Autodesk Fusion 360 part; units mm, degrees
note: some values were not read from the file. Set by a fixed rule: which sketch regions a step uses.
(part 17 of 59)
  spline S95 degree 5 poles (2.1183, -16.4679) (2.1183, -16.468) (2.1183, -16.4682) (2.1183, -16.4685) (2.1184, -16.469) (2.1184, -16.4698) (2.1185, -16.4706) (2.1186, -16.4716) (2.1187, -16.4727) (2.1188, -16.4739) (2.1189, -16.4752) (2.1191, -16.4766) (2.1192, -16.4781) (2.1194, -16.4798) (2.1196, -16.4815) (2.1198, -16.4833) (2.12, -16.4852) (2.1202, -16.4873) (2.1204, -16.4894) (2.1207, -16.4916) (2.121, -16.4939) (2.1212, -16.4963) (2.1215, -16.4989) (2.1219, -16.5015) (2.1222, -16.5041) (2.1225, -16.5069) (2.1229, -16.5098) (2.1233, -16.5128) (2.1237, -16.5158) (2.1241, -16.5189) (2.1245, -16.5222) (2.125, -16.5255) (2.1254, -16.5289) (2.1259, -16.5323) (2.1264, -16.5359) (2.127, -16.5395) (2.1275, -16.5432) (2.1281, -16.547) (2.1286, -16.5509) (2.1292, -16.5549) (2.1299, -16.5589) (2.1305, -16.563) (2.1312, -16.5672) (2.1318, -16.5714) (2.1325, -16.5758) (2.1332, -16.5802) (2.134, -16.5847) (2.1347, -16.5892) (2.1355, -16.5938) (2.1363, -16.5985) (2.1371, -16.6033) (2.138, -16.6081) (2.1388, -16.6131) (2.1397, -16.618) (2.1406, -16.6231) (2.1415, -16.6282) (2.1424, -16.6334) (2.1434, -16.6386) (2.1444, -16.6439) (2.1454, -16.6493) (2.1464, -16.6547) (2.1475, -16.6602) (2.1485, -16.6658) (2.1496, -16.6714) (2.1507, -16.6771) (2.1519, -16.6829) (2.153, -16.6887) (2.1542, -16.6946) (2.1554, -16.7005) (2.1567, -16.7065) (2.1579, -16.7126) (2.1592, -16.7187) (2.1605, -16.7249) (2.1618, -16.7311) (2.1631, -16.7374) (2.1645, -16.7438) (2.1659, -16.7502) (2.1673, -16.7567) (2.1687, -16.7632) (2.1702, -16.7698) (2.1716, -16.7764) (2.1731, -16.7831) (2.1747, -16.7899) (2.1762, -16.7967) (2.1778, -16.8035) (2.1794, -16.8104) (2.181, -16.8174) (2.1827, -16.8244) (2.1843, -16.8314) (2.186, -16.8386) (2.1877, -16.8457) (2.1895, -16.8529) (2.1912, -16.8602) (2.193, -16.8675) (2.1948, -16.8749) (2.1967, -16.8823) (2.1985, -16.8898) (2.2004, -16.8973) (2.2023, -16.9049) (2.2043, -16.9125) (2.2062, -16.9202) (2.2082, -16.9279) (2.2102, -16.9356) (2.2123, -16.9434) (2.2143, -16.9513) (2.2164, -16.9592) (2.2185, -16.9671) (2.2207, -16.9751) (2.2228, -16.9832) (2.225, -16.9912) (2.2272, -16.9994) (2.2295, -17.0075) (2.2317, -17.0158) (2.234, -17.024) (2.2363, -17.0323) (2.2387, -17.0407) (2.241, -17.0491) (2.2434, -17.0575) (2.2458, -17.066) (2.2483, -17.0745) (2.2508, -17.083) (2.2533, -17.0917) (2.2558, -17.1003) (2.2583, -17.109) (2.2609, -17.1177) (2.2635, -17.1265) (2.2661, -17.1353) (2.2688, -17.1441) (2.2714, -17.153) (2.2741, -17.1619) (2.2769, -17.1709) (2.2796, -17.1799) (2.2824, -17.189) (2.2852, -17.1981) (2.288, -17.2072) (2.2909, -17.2163) (2.2938, -17.2255) (2.2967, -17.2348) (2.2996, -17.2441) (2.3026, -17.2534) (2.3056, -17.2627) (2.3086, -17.2721) (2.3117, -17.2815) (2.3147, -17.291) (2.3178, -17.3005) (2.321, -17.31) (2.3241, -17.3196) (2.3273, -17.3292) (2.3305, -17.3388) (2.3337, -17.3485) (2.337, -17.3582) (2.3403, -17.368) (2.3436, -17.3777) (2.3469, -17.3875) (2.3503, -17.3974) (2.3537, -17.4073) (2.3571, -17.4172) (2.3606, -17.4271) (2.364, -17.4371) (2.3675, -17.4471) (2.3711, -17.4572) (2.3746, -17.4673) (2.3782, -17.4774) (2.3818, -17.4875) (2.3855, -17.4977) (2.3891, -17.5079) (2.3928, -17.5182) (2.3965, -17.5284) (2.4003, -17.5388) (2.4041, -17.5491) (2.4079, -17.5595) (2.4117, -17.5699) (2.4156, -17.5803) (2.4194, -17.5907) (2.4234, -17.6012) (2.4273, -17.6118) (2.4313, -17.6223) (2.4353, -17.6329) (2.4393, -17.6435) (2.4433, -17.6541) (2.4474, -17.6648) (2.4515, -17.6755) (2.4557, -17.6862) (2.4598, -17.697) (2.464, -17.7078) (2.4682, -17.7186) (2.4725, -17.7294) (2.4767, -17.7403) (2.481, -17.7512) (2.4854, -17.7621) (2.4897, -17.7731) (2.4941, -17.7841) (2.4985, -17.7951) (2.503, -17.8061) (2.5074, -17.8172) (2.5119, -17.8283) (2.5165, -17.8394) (2.521, -17.8506) (2.5256, -17.8617) (2.5302, -17.8729) (2.5348, -17.8841) (2.5395, -17.8954) (2.5442, -17.9067) (2.5489, -17.918) (2.5537, -17.9293) (2.5584, -17.9407) (2.5632, -17.952) (2.5681, -17.9634) (2.5729, -17.9749) (2.5778, -17.9863) (2.5827, -17.9978) (2.5877, -18.0093) (2.5927, -18.0208) (2.5977, -18.0324) (2.6027, -18.0439) (2.6077, -18.0555) (2.6128, -18.0672) (2.6179, -18.0788) (2.6231, -18.0905) (2.6283, -18.1022) (2.6335, -18.1139) (2.6387, -18.1256) (2.6439, -18.1374) (2.6492, -18.1492) (2.6545, -18.161) (2.6599, -18.1728) (2.6653, -18.1847) (2.6707, -18.1966) (2.6761, -18.2085) (2.6815, -18.2204) (2.687, -18.2323) (2.6925, -18.2443) (2.6981, -18.2563) (2.7036, -18.2683) (2.7092, -18.2803) (2.7149, -18.2924) (2.7205, -18.3044) (2.7262, -18.3165) (2.7319, -18.3287) (2.7376, -18.3408) (2.7434, -18.353) (2.748, -18.3627) (2.7515, -18.37) (2.7539, -18.3749) (2.755, -18.3773) knots 0 0 0 0 0 0 0.00416667 0.00833333 0.0125 0.01666667 0.02083333 0.025 0.02916667 0.03333333 0.0375 0.04166667 0.04583333 0.05 0.05416667 0.05833333 0.0625 0.06666667 0.07083333 0.075 0.07916667 0.08333333 0.0875 0.09166667 0.09583333 0.1 0.10416667 0.10833333 0.1125 0.11666667 0.12083333 0.125 0.12916667 0.13333333 0.1375 0.14166667 0.14583333 0.15 0.15416667 0.15833333 0.1625 0.16666667 0.17083333 0.175 0.17916667 0.18333333 0.1875 0.19166667 0.19583333 0.2 0.20416667 0.20833333 0.2125 0.21666667 0.22083333 0.225 0.22916667 0.23333333 0.2375 0.24166667 0.24583333 0.25 0.25416667 0.25833333 0.2625 0.26666667 0.27083333 0.275 0.27916667 0.28333333 0.2875 0.29166667 0.29583333 0.3 0.30416667 0.30833333 0.3125 0.31666667 0.32083333 0.325 0.32916667 0.33333333 0.3375 0.34166667 0.34583333 0.35 0.35416667 0.35833333 0.3625 0.36666667 0.37083333 0.375 0.37916667 0.38333333 0.3875 0.39166667 0.39583333 0.4 0.40416667 0.40833333 0.4125 0.41666667 0.42083333 0.425 0.42916667 0.43333333 0.4375 0.44166667 0.44583333 0.45 0.45416667 0.45833333 0.4625 0.46666667 0.47083333 0.475 0.47916667 0.48333333 0.4875 0.49166667 0.49583333 0.5 0.50416667 0.50833333 0.5125 0.51666667 0.52083333 0.525 0.52916667 0.53333333 0.5375 0.54166667 0.54583333 0.55 0.55416667 0.55833333 0.5625 0.56666667 0.57083333 0.575 0.57916667 0.58333333 0.5875 0.59166667 0.59583333 0.6 0.60416667 0.60833333 0.6125 0.61666667 0.62083333 0.625 0.62916667 0.63333333 0.6375 0.64166667 0.64583333 0.65 0.65416667 0.65833333 0.6625 0.66666667 0.67083333 0.675 0.67916667 0.68333333 0.6875 0.69166667 0.69583333 0.7 0.70416667 0.70833333 0.7125 0.71666667 0.72083333 0.725 0.72916667 0.73333333 0.7375 0.74166667 0.74583333 0.75 0.75416667 0.75833333 0.7625 0.76666667 0.77083333 0.775 0.77916667 0.78333333 0.7875 0.79166667 0.79583333 0.8 0.80416667 0.80833333 0.8125 0.81666667 0.82083333 0.825 0.82916667 0.83333333 0.8375 0.84166667 0.84583333 0.85 0.85416667 0.85833333 0.8625 0.86666667 0.87083333 0.875 0.87916667 0.88333333 0.8875 0.89166667 0.89583333 0.9 0.90416667 0.90833333 0.9125 0.91666667 0.92083333 0.925 0.92916667 0.93333333 0.9375 0.94166667 0.94583333 0.95 0.95416667 0.95833333 0.9625 0.96666667 0.97083333 0.975 0.97916667 0.98333333 0.9875 0.99166667 0.99583333 1 1 1 1 1 1
  line L207 (15.3132, -12.1806) -> (15.3128, -12.1799)
  line L208 (27.6109, 20.5125) -> (27.8937, 20.5945)
  line L209 (26.1461, 25.1495) -> (26.1453, 25.1491)
  arc A105 (26.5997, -3.4204) -> (27.0873, -2.5758) centre (0, 12.5) ccw
  arc A106 (12.1618, -16.0147) -> (13.0527, -15.6181) centre (0, 12.5) ccw
  line L210 (27.8937, 20.5945) -> (27.8945, 20.5948)
  arc A107 (24.7898, -6.1136) -> (25.363, -5.3246) centre (0, 12.5) ccw
  line L211 (-22.1904, 31.2406) -> (-22.1898, 31.2401)
  line L212 (-9.7471, -14.5473) -> (-9.8469, -14.8243)
  arc A108 (17.6281, -10.2115) -> (18.5501, -9.4649) centre (0, 12.5) ccw
  line L213 (-9.8469, -14.8243) -> (-9.8472, -14.8251)
  line L214 (-22.1898, 31.2401) -> (-21.9649, 31.0501)
  line L215 (-13.7171, -13.1012) -> (-13.578, -12.8417)
  spline S96 degree 5 poles (28.1181, 25.5527) (28.1154, 25.5525) (28.11, 25.5521) (28.1019, 25.5515) (28.0911, 25.5506) (28.0777, 25.5495) (28.0644, 25.5484) (28.051, 25.5473) (28.0377, 25.5462) (28.0244, 25.5451) (28.0112, 25.5439) (27.9979, 25.5427) (27.9848, 25.5415) (27.9716, 25.5404) (27.9585, 25.5391) (27.9454, 25.5379) (27.9323, 25.5367) (27.9193, 25.5354) (27.9063, 25.5342) (27.8934, 25.5329) (27.8805, 25.5316) (27.8676, 25.5303) (27.8547, 25.529) (27.8419, 25.5276) (27.8291, 25.5263) (27.8164, 25.5249) (27.8037, 25.5236) (27.791, 25.5222) (27.7784, 25.5208) (27.7658, 25.5194) (27.7532, 25.518) (27.7406, 25.5165) (27.7281, 25.5151) (27.7157, 25.5136) (27.7032, 25.5122) (27.6908, 25.5107) (27.6785, 25.5092) (27.6661, 25.5077) (27.6539, 25.5062) (27.6416, 25.5047) (27.6294, 25.5031) (27.6172, 25.5016) (27.605, 25.5) (27.5929, 25.4984) (27.5809, 25.4968) (27.5688, 25.4952) (27.5568, 25.4936) (27.5449, 25.492) (27.5329, 25.4904) (27.521, 25.4887) (27.5092, 25.4871) (27.4974, 25.4854) (27.4856, 25.4838) (27.4738, 25.4821) (27.4621, 25.4804) (27.4505, 25.4787) (27.4388, 25.477) (27.4273, 25.4752) (27.4157, 25.4735) (27.4042, 25.4718) (27.3927, 25.47) (27.3813, 25.4682) (27.3699, 25.4665) (27.3585, 25.4647) (27.3472, 25.4629) (27.3359, 25.4611) (27.3247, 25.4593) (27.3135, 25.4574) (27.3023, 25.4556) (27.2912, 25.4538) (27.2801, 25.4519) (27.2691, 25.4501) (27.2581, 25.4482) (27.2471, 25.4463) (27.2362, 25.4445) (27.2253, 25.4426) (27.2145, 25.4407) (27.2037, 25.4388) (27.1929, 25.4368) (27.1822, 25.4349) (27.1715, 25.433) (27.1609, 25.4311) (27.1503, 25.4291) (27.1397, 25.4272) (27.1292, 25.4252) (27.1188, 25.4232) (27.1083, 25.4213) (27.0979, 25.4193) (27.0876, 25.4173) (27.0773, 25.4153) (27.0671, 25.4133) (27.0568, 25.4113) (27.0467, 25.4093) (27.0365, 25.4072) (27.0265, 25.4052) (27.0164, 25.4032) (27.0064, 25.4011) (26.9965, 25.3991) (26.9866, 25.3971) (26.9767, 25.395) (26.9669, 25.3929) (26.9571, 25.3909) (26.9474, 25.3888) (26.9377, 25.3867) (26.9281, 25.3847) (26.9185, 25.3826) (26.9089, 25.3805) (26.8994, 25.3784) (26.89, 25.3763) (26.8806, 25.3742) (26.8712, 25.3721) (26.8619, 25.37) (26.8526, 25.3679) (26.8434, 25.3658) (26.8342, 25.3636) (26.8251, 25.3615) (26.816, 25.3594) (26.8069, 25.3573) (26.798, 25.3551) (26.789, 25.353) (26.7801, 25.3509) (26.7713, 25.3487) (26.7625, 25.3466) (26.7537, 25.3445) (26.7451, 25.3423) (26.7364, 25.3402) (26.7278, 25.338) (26.7193, 25.3359) (26.7108, 25.3337) (26.7023, 25.3316) (26.6939, 25.3294) (26.6856, 25.3273) (26.6773, 25.3251) (26.669, 25.323) (26.6608, 25.3208) (26.6527, 25.3187) (26.6446, 25.3166) (26.6365, 25.3144) (26.6286, 25.3123) (26.6206, 25.3101) (26.6127, 25.308) (26.6049, 25.3058) (26.5971, 25.3037) (26.5894, 25.3016) (26.5817, 25.2994) (26.5741, 25.2973) (26.5665, 25.2952) (26.559, 25.293) (26.5516, 25.2909) (26.5442, 25.2888) (26.5368, 25.2867) (26.5296, 25.2845) (26.5223, 25.2824) (26.5151, 25.2803) (26.508, 25.2782) (26.5009, 25.2761) (26.4939, 25.274) (26.487, 25.272) (26.4801, 25.2699) (26.4733, 25.2678) (26.4665, 25.2657) (26.4598, 25.2637) (26.4531, 25.2616) (26.4465, 25.2596) (26.4399, 25.2575) (26.4335, 25.2555) (26.427, 25.2534) (26.4207, 25.2514) (26.4144, 25.2494) (26.4081, 25.2474) (26.4019, 25.2454) (26.3958, 25.2434) (26.3897, 25.2414) (26.3837, 25.2395) (26.3778, 25.2375) (26.3719, 25.2356) (26.3661, 25.2336) (26.3604, 25.2317) (26.3547, 25.2298) (26.3491, 25.2279) (26.3435, 25.226) (26.338, 25.2241) (26.3326, 25.2222) (26.3273, 25.2204) (26.322, 25.2185) (26.3167, 25.2167) (26.3116, 25.2149) (26.3065, 25.2131) (26.3015, 25.2113) (26.2965, 25.2095) (26.2916, 25.2077) (26.2868, 25.206) (26.282, 25.2043) (26.2774, 25.2026) (26.2728, 25.2009) (26.2682, 25.1992) (26.2638, 25.1975) (26.2594, 25.1959) (26.255, 25.1943) (26.2508, 25.1927) (26.2466, 25.1911) (26.2425, 25.1895) (26.2385, 25.188) (26.2345, 25.1864) (26.2307, 25.1849) (26.2269, 25.1834) (26.2231, 25.182) (26.2195, 25.1806) (26.2159, 25.1791) (26.2124, 25.1778) (26.209, 25.1764) (26.2057, 25.175) (26.2024, 25.1737) (26.1993, 25.1724) (26.1962, 25.1712) (26.1932, 25.1699) (26.1903, 25.1687) (26.1874, 25.1676) (26.1847, 25.1664) (26.182, 25.1653) (26.1794, 25.1642) (26.1769, 25.1631) (26.1745, 25.1621) (26.1722, 25.1611) (26.17, 25.1602) (26.1678, 25.1592) (26.1658, 25.1583) (26.1638, 25.1575) (26.1619, 25.1567) (26.1602, 25.1559) (26.1585, 25.1551) (26.1569, 25.1544) (26.1554, 25.1538) (26.154, 25.1531) (26.1527, 25.1526) (26.1515, 25.152) (26.1504, 25.1515) (26.1495, 25.151) (26.1486, 25.1506) (26.1478, 25.1503) (26.1471, 25.15) (26.1467, 25.1497) (26.1464, 25.1496) (26.1462, 25.1495) (26.1461, 25.1495) knots -1 -1 -1 -1 -1 -1 -0.99583333 -0.99166667 -0.9875 -0.98333333 -0.97916667 -0.975 -0.97083333 -0.96666667 -0.9625 -0.95833333 -0.95416667 -0.95 -0.94583333 -0.94166667 -0.9375 -0.93333333 -0.92916667 -0.925 -0.92083333 -0.91666667 -0.9125 -0.90833333 -0.90416667 -0.9 -0.89583333 -0.89166667 -0.8875 -0.88333333 -0.87916667 -0.875 -0.87083333 -0.86666667 -0.8625 -0.85833333 -0.85416667 -0.85 -0.84583333 -0.84166667 -0.8375 -0.83333333 -0.82916667 -0.825 -0.82083333 -0.81666667 -0.8125 -0.80833333 -0.80416667 -0.8 -0.79583333 -0.79166667 -0.7875 -0.78333333 -0.77916667 -0.775 -0.77083333 -0.76666667 -0.7625 -0.75833333 -0.75416667 -0.75 -0.74583333 -0.74166667 -0.7375 -0.73333333 -0.72916667 -0.725 -0.72083333 -0.71666667 -0.7125 -0.70833333 -0.70416667 -0.7 -0.69583333 -0.69166667 -0.6875 -0.68333333 -0.67916667 -0.675 -0.67083333 -0.66666667 -0.6625 -0.65833333 -0.65416667 -0.65 -0.64583333 -0.64166667 -0.6375 -0.63333333 -0.62916667 -0.625 -0.62083333 -0.61666667 -0.6125 -0.60833333 -0.60416667 -0.6 -0.59583333 -0.59166667 -0.5875 -0.58333333 -0.57916667 -0.575 -0.57083333 -0.56666667 -0.5625 -0.55833333 -0.55416667 -0.55 -0.54583333 -0.54166667 -0.5375 -0.53333333 -0.52916667 -0.525 -0.52083333 -0.51666667 -0.5125 -0.50833333 -0.50416667 -0.5 -0.49583333 -0.49166667 -0.4875 -0.48333333 -0.47916667 -0.475 -0.47083333 -0.46666667 -0.4625 -0.45833333 -0.45416667 -0.45 -0.44583333 -0.44166667 -0.4375 -0.43333333 -0.42916667 -0.425 -0.42083333 -0.41666667 -0.4125 -0.40833333 -0.40416667 -0.4 -0.39583333 -0.39166667 -0.3875 -0.38333333 -0.37916667 -0.375 -0.37083333 -0.36666667 -0.3625 -0.35833333 -0.35416667 -0.35 -0.34583333 -0.34166667 -0.3375 -0.33333333 -0.32916667 -0.325 -0.32083333 -0.31666667 -0.3125 -0.30833333 -0.30416667 -0.3 -0.29583333 -0.29166667 -0.2875 -0.28333333 -0.27916667 -0.275 -0.27083333 -0.26666667 -0.2625 -0.25833333 -0.25416667 -0.25 -0.24583333 -0.24166667 -0.2375 -0.23333333 -0.22916667 -0.225 -0.22083333 -0.21666667 -0.2125 -0.20833333 -0.20416667 -0.2 -0.19583333 -0.19166667 -0.1875 -0.18333333 -0.17916667 -0.175 -0.17083333 -0.16666667 -0.1625 -0.15833333 -0.15416667 -0.15 -0.14583333 -0.14166667 -0.1375 -0.13333333 -0.12916667 -0.125 -0.12083333 -0.11666667 -0.1125 -0.10833333 -0.10416667 -0.1 -0.09583333 -0.09166667 -0.0875 -0.08333333 -0.07916667 -0.075 -0.07083333 -0.06666667 -0.0625 -0.05833333 -0.05416667 -0.05 -0.04583333 -0.04166667 -0.0375 -0.03333333 -0.02916667 -0.025 -0.02083333 -0.01666667 -0.0125 -0.00833333 -0.00416667 0 0 0 0 0 0
  spline S97 degree 5 poles (30.2174, 19.4214) (30.2148, 19.4218) (30.2094, 19.4225) (30.2014, 19.4236) (30.1907, 19.425) (30.1773, 19.4267) (30.164, 19.4284) (30.1507, 19.4301) (30.1375, 19.4317) (30.1242, 19.4334) (30.111, 19.435) (30.0979, 19.4366) (30.0847, 19.4382) (30.0716, 19.4398) (30.0585, 19.4413) (30.0455, 19.4428) (30.0324, 19.4443) (30.0194, 19.4458) (30.0065, 19.4473) (29.9935, 19.4487) (29.9806, 19.4501) (29.9678, 19.4516) (29.9549, 19.4529) (29.9421, 19.4543) (29.9293, 19.4556) (29.9166, 19.457) (29.9039, 19.4583) (29.8912, 19.4596) (29.8785, 19.4608) (29.8659, 19.4621) (29.8533, 19.4633) (29.8407, 19.4645) (29.8282, 19.4657) (29.8157, 19.4669) (29.8032, 19.468) (29.7908, 19.4691) (29.7784, 19.4702) (29.766, 19.4713) (29.7537, 19.4724) (29.7414, 19.4735) (29.7291, 19.4745) (29.7169, 19.4755) (29.7047, 19.4765) (29.6925, 19.4775) (29.6803, 19.4784) (29.6682, 19.4794) (29.6562, 19.4803) (29.6441, 19.4812) (29.6321, 19.4821) (29.6201, 19.483) (29.6082, 19.4838) (29.5963, 19.4846) (29.5844, 19.4855) (29.5726, 19.4863) (29.5608, 19.487) (29.549, 19.4878) (29.5373, 19.4885) (29.5256, 19.4892) (29.514, 19.49) (29.5023, 19.4906) (29.4907, 19.4913) (29.4792, 19.492) (29.4677, 19.4926) (29.4562, 19.4932) (29.4447, 19.4938) (29.4333, 19.4944) (29.422, 19.495) (29.4106, 19.4955) (29.3993, 19.496) (29.3881, 19.4965) (29.3768, 19.497) (29.3657, 19.4975) (29.3545, 19.498) (29.3434, 19.4984) (29.3323, 19.4989) (29.3213, 19.4993) (29.3103, 19.4997) (29.2993, 19.5001) (29.2884, 19.5004) (29.2775, 19.5008) (29.2667, 19.5011) (29.2559, 19.5014) (29.2451, 19.5017) (29.2344, 19.502) (29.2237, 19.5023) (29.213, 19.5025) (29.2024, 19.5028) (29.1919, 19.503) (29.1813, 19.5032) (29.1708, 19.5034) (29.1604, 19.5035) (29.15, 19.5037) (29.1396, 19.5038) (29.1293, 19.504) (29.119, 19.5041) (29.1088, 19.5042) (29.0986, 19.5043) (29.0884, 19.5043) (29.0783, 19.5044) (29.0682, 19.5044) (29.0582, 19.5045) (29.0482, 19.5045) (29.0383, 19.5045) (29.0284, 19.5045) (29.0185, 19.5044) (29.0087, 19.5044) (28.9989, 19.5043) (28.9892, 19.5043) (28.9795, 19.5042) (28.9698, 19.5041) (28.9602, 19.504) (28.9507, 19.5038) (28.9412, 19.5037) (28.9317, 19.5036) (28.9223, 19.5034) (28.9129, 19.5032) (28.9036, 19.503) (28.8943, 19.5028) (28.8851, 19.5026) (28.8759, 19.5024) (28.8668, 19.5021) (28.8577, 19.5019) (28.8486, 19.5016) (28.8396, 19.5014) (28.8307, 19.5011) (28.8218, 19.5008) (28.8129, 19.5005) (28.8041, 19.5001) (28.7953, 19.4998) (28.7866, 19.4995) (28.778, 19.4991) (28.7694, 19.4987) (28.7608, 19.4984) (28.7523, 19.498) (28.7438, 19.4976) (28.7354, 19.4972) (28.727, 19.4968) (28.7187, 19.4963) (28.7105, 19.4959) (28.7023, 19.4954) (28.6941, 19.495) (28.686, 19.4945) (28.678, 19.494) (28.67, 19.4936) (28.662, 19.4931) (28.6541, 19.4926) (28.6463, 19.4921) (28.6385, 19.4915) (28.6307, 19.491) (28.6231, 19.4905) (28.6154, 19.4899) (28.6079, 19.4894) (28.6004, 19.4888) (28.5929, 19.4882) (28.5855, 19.4877) (28.5781, 19.4871) (28.5709, 19.4865) (28.5636, 19.4859) (28.5564, 19.4853) (28.5493, 19.4847) (28.5423, 19.4841) (28.5353, 19.4835) (28.5283, 19.4828) (28.5214, 19.4822) (28.5146, 19.4816) (28.5078, 19.4809) (28.5011, 19.4803) (28.4945, 19.4796) (28.4879, 19.4789) (28.4814, 19.4783) (28.4749, 19.4776) (28.4685, 19.4769) (28.4622, 19.4763) (28.4559, 19.4756) (28.4497, 19.4749) (28.4435, 19.4742) (28.4374, 19.4735) (28.4314, 19.4728) (28.4255, 19.4721) (28.4196, 19.4714) (28.4137, 19.4707) (28.408, 19.47) (28.4023, 19.4693) (28.3966, 19.4686) (28.3911, 19.4679) (28.3856, 19.4672) (28.3802, 19.4665) (28.3748, 19.4658) (28.3695, 19.4651) (28.3643, 19.4644) (28.3592, 19.4637) (28.3541, 19.463) (28.3491, 19.4623) (28.3442, 19.4616) (28.3393, 19.4609) (28.3345, 19.4602) (28.3298, 19.4595) (28.3252, 19.4588) (28.3206, 19.4581) (28.3161, 19.4574) (28.3117, 19.4568) (28.3074, 19.4561) (28.3031, 19.4554) (28.2989, 19.4547) (28.2948, 19.4541) (28.2908, 19.4534) (28.2868, 19.4528) (28.283, 19.4521) (28.2792, 19.4515) (28.2755, 19.4508) (28.2719, 19.4502) (28.2683, 19.4496) (28.2649, 19.449) (28.2615, 19.4484) (28.2582, 19.4478) (28.255, 19.4472) (28.2519, 19.4466) (28.2489, 19.4461) (28.246, 19.4455) (28.2431, 19.445) (28.2404, 19.4445) (28.2377, 19.4439) (28.2351, 19.4434) (28.2327, 19.4429) (28.2303, 19.4425) (28.228, 19.442) (28.2258, 19.4416) (28.2237, 19.4411) (28.2217, 19.4407) (28.2198, 19.4403) (28.218, 19.4399) (28.2163, 19.4396) (28.2147, 19.4392) (28.2132, 19.4389) (28.2118, 19.4386) (28.2106, 19.4383) (28.2094, 19.4381) (28.2083, 19.4378) (28.2074, 19.4376) (28.2065, 19.4374) (28.2058, 19.4372) (28.2053, 19.4371) (28.205, 19.437) (28.2048, 19.437) (28.2047, 19.437) knots -1 -1 -1 -1 -1 -1 -0.99583333 -0.99166667 -0.9875 -0.98333333 -0.97916667 -0.975 -0.97083333 -0.96666667 -0.9625 -0.95833333 -0.95416667 -0.95 -0.94583333 -0.94166667 -0.9375 -0.93333333 -0.92916667 -0.925 -0.92083333 -0.91666667 -0.9125 -0.90833333 -0.90416667 -0.9 -0.89583333 -0.89166667 -0.8875 -0.88333333 -0.87916667 -0.875 -0.87083333 -0.86666667 -0.8625 -0.85833333 -0.85416667 -0.85 -0.84583333 -0.84166667 -0.8375 -0.83333333 -0.82916667 -0.825 -0.82083333 -0.81666667 -0.8125 -0.80833333 -0.80416667 -0.8 -0.79583333 -0.79166667 -0.7875 -0.78333333 -0.77916667 -0.775 -0.77083333 -0.76666667 -0.7625 -0.75833333 -0.75416667 -0.75 -0.74583333 -0.74166667 -0.7375 -0.73333333 -0.72916667 -0.725 -0.72083333 -0.71666667 -0.7125 -0.70833333 -0.70416667 -0.7 -0.69583333 -0.69166667 -0.6875 -0.68333333 -0.67916667 -0.675 -0.67083333 -0.66666667 -0.6625 -0.65833333 -0.65416667 -0.65 -0.64583333 -0.64166667 -0.6375 -0.63333333 -0.62916667 -0.625 -0.62083333 -0.61666667 -0.6125 -0.60833333 -0.60416667 -0.6 -0.59583333 -0.59166667 -0.5875 -0.58333333 -0.57916667 -0.575 -0.57083333 -0.56666667 -0.5625 -0.55833333 -0.55416667 -0.55 -0.54583333 -0.54166667 -0.5375 -0.53333333 -0.52916667 -0.525 -0.52083333 -0.51666667 -0.5125 -0.50833333 -0.50416667 -0.5 -0.49583333 -0.49166667 -0.4875 -0.48333333 -0.47916667 -0.475 -0.47083333 -0.46666667 -0.4625 -0.45833333 -0.45416667 -0.45 -0.44583333 -0.44166667 -0.4375 -0.43333333 -0.42916667 -0.425 -0.42083333 -0.41666667 -0.4125 -0.40833333 -0.40416667 -0.4 -0.39583333 -0.39166667 -0.3875 -0.38333333 -0.37916667 -0.375 -0.37083333 -0.36666667 -0.3625 -0.35833333 -0.35416667 -0.35 -0.34583333 -0.34166667 -0.3375 -0.33333333 -0.32916667 -0.325 -0.32083333 -0.31666667 -0.3125 -0.30833333 -0.30416667 -0.3 -0.29583333 -0.29166667 -0.2875 -0.28333333 -0.27916667 -0.275 -0.27083333 -0.26666667 -0.2625 -0.25833333 -0.25416667 -0.25 -0.24583333 -0.24166667 -0.2375 -0.23333333 -0.22916667 -0.225 -0.22083333 -0.21666667 -0.2125 -0.20833333 -0.20416667 -0.2 -0.19583333 -0.19166667 -0.1875 -0.18333333 -0.17916667 -0.175 -0.17083333 -0.16666667 -0.1625 -0.15833333 -0.15416667 -0.15 -0.14583333 -0.14166667 -0.1375 -0.13333333 -0.12916667 -0.125 -0.12083333 -0.11666667 -0.1125 -0.10833333 -0.10416667 -0.1 -0.09583333 -0.09166667 -0.0875 -0.08333333 -0.07916667 -0.075 -0.07083333 -0.06666667 -0.0625 -0.05833333 -0.05416667 -0.05 -0.04583333 -0.04166667 -0.0375 -0.03333333 -0.02916667 -0.025 -0.02083333 -0.01666667 -0.0125 -0.00833333 -0.00416667 0 0 0 0 0 0
  line L216 (-12.6491, -13.6453) -> (-12.6495, -13.6461)
  line L217 (-22.9441, 30.3086) -> (-22.9448, 30.3091)
  line L218 (-13.7175, -13.1019) -> (-13.7171, -13.1012)
  spline S98 degree 5 poles (25.6019, 26.2175) (25.602, 26.2175) (25.6022, 26.2176) (25.6025, 26.2178) (25.6029, 26.218) (25.6036, 26.2184) (25.6043, 26.2188) (25.6052, 26.2193) (25.6061, 26.2198) (25.6072, 26.2204) (25.6083, 26.221) (25.6096, 26.2217) (25.6109, 26.2225) (25.6123, 26.2233) (25.6138, 26.2242) (25.6154, 26.2251) (25.6171, 26.2261) (25.6188, 26.2271) (25.6207, 26.2282) (25.6226, 26.2293) (25.6246, 26.2305) (25.6267, 26.2317) (25.6289, 26.233) (25.6311, 26.2344) (25.6334, 26.2358) (25.6358, 26.2372) (25.6383, 26.2387) (25.6409, 26.2403) (25.6435, 26.2419) (25.6462, 26.2435) (25.6489, 26.2452) (25.6518, 26.247) (25.6547, 26.2488) (25.6577, 26.2506) (25.6607, 26.2526) (25.6638, 26.2545) (25.667, 26.2565) (25.6702, 26.2586) (25.6735, 26.2607) (25.6769, 26.2628) (25.6803, 26.265) (25.6838, 26.2673) (25.6874, 26.2696) (25.691, 26.2719) (25.6947, 26.2743) (25.6984, 26.2768) (25.7022, 26.2793) (25.706, 26.2818) (25.71, 26.2844) (25.7139, 26.287) (25.718, 26.2897) (25.722, 26.2925) (25.7262, 26.2952) (25.7304, 26.2981) (25.7346, 26.3009) (25.7389, 26.3039) (25.7432, 26.3068) (25.7476, 26.3098) (25.7521, 26.3129) (25.7566, 26.316) (25.7612, 26.3192) (25.7658, 26.3224) (25.7704, 26.3256) (25.7751, 26.3289) (25.7799, 26.3322) (25.7847, 26.3356) (25.7895, 26.339) (25.7944, 26.3425) (25.7993, 26.346) (25.8043, 26.3496) (25.8093, 26.3532) (25.8144, 26.3568) (25.8195, 26.3605) (25.8247, 26.3643) (25.8299, 26.3681) (25.8352, 26.3719) (25.8405, 26.3758) (25.8458, 26.3797) (25.8512, 26.3836) (25.8566, 26.3876) (25.8621, 26.3917) (25.8676, 26.3958) (25.8731, 26.3999) (25.8787, 26.4041) (25.8843, 26.4083) (25.89, 26.4126) (25.8957, 26.4169) (25.9014, 26.4213) (25.9072, 26.4257) (25.913, 26.4301) (25.9188, 26.4346) (25.9247, 26.4391) (25.9306, 26.4437) (25.9366, 26.4483) (25.9426, 26.4529) (25.9486, 26.4576) (25.9547, 26.4624) (25.9608, 26.4672) (25.9669, 26.472) (25.9731, 26.4769) (25.9793, 26.4818) (25.9855, 26.4867) (25.9918, 26.4917) (25.9981, 26.4967) (26.0044, 26.5018) (26.0108, 26.5069) (26.0172, 26.5121) (26.0236, 26.5173) (26.0301, 26.5225) (26.0366, 26.5278) (26.0431, 26.5332) (26.0497, 26.5385) (26.0563, 26.5439) (26.0629, 26.5494) (26.0695, 26.5549) (26.0762, 26.5604) (26.0829, 26.566) (26.0896, 26.5716) (26.0964, 26.5772) (26.1032, 26.5829) (26.11, 26.5887) (26.1168, 26.5945) (26.1237, 26.6003) (26.1306, 26.6061) (26.1375, 26.612) (26.1445, 26.618) (26.1515, 26.6239) (26.1585, 26.63) (26.1655, 26.636) (26.1726, 26.6421) (26.1796, 26.6483) (26.1868, 26.6544) (26.1939, 26.6607) (26.201, 26.6669) (26.2082, 26.6732) (26.2154, 26.6796) (26.2227, 26.6859) (26.2299, 26.6924) (26.2372, 26.6988) (26.2445, 26.7053) (26.2518, 26.7119) (26.2592, 26.7184) (26.2665, 26.725) (26.2739, 26.7317) (26.2813, 26.7384) (26.2888, 26.7451) (26.2962, 26.7519) (26.3037, 26.7587) (26.3112, 26.7656) (26.3188, 26.7724) (26.3263, 26.7794) (26.3339, 26.7863) (26.3414, 26.7933) (26.3491, 26.8004) (26.3567, 26.8075) (26.3643, 26.8146) (26.372, 26.8217) (26.3797, 26.8289) (26.3874, 26.8362) (26.3951, 26.8435) (26.4029, 26.8508) (26.4106, 26.8581) (26.4184, 26.8655) (26.4262, 26.8729) (26.434, 26.8804) (26.4419, 26.8879) (26.4497, 26.8954) (26.4576, 26.903) (26.4655, 26.9106) (26.4734, 26.9183) (26.4813, 26.926) (26.4893, 26.9337) (26.4972, 26.9415) (26.5052, 26.9493) (26.5132, 26.9571) (26.5212, 26.965) (26.5292, 26.9729) (26.5373, 26.9809) (26.5453, 26.9889) (26.5534, 26.9969) (26.5615, 27.005) (26.5696, 27.0131) (26.5777, 27.0212) (26.5858, 27.0294) (26.594, 27.0376) (26.6022, 27.0459) (26.6103, 27.0541) (26.6185, 27.0625) (26.6267, 27.0708) (26.635, 27.0792) (26.6432, 27.0877) (26.6514, 27.0961) (26.6597, 27.1046) (26.668, 27.1132) (26.6763, 27.1218) (26.6846, 27.1304) (26.6929, 27.139) (26.7012, 27.1477) (26.7096, 27.1565) (26.7179, 27.1652) (26.7263, 27.174) (26.7347, 27.1829) (26.7431, 27.1917) (26.7515, 27.2006) (26.7599, 27.2096) (26.7683, 27.2186) (26.7767, 27.2276) (26.7852, 27.2366) (26.7937, 27.2457) (26.8021, 27.2549) (26.8106, 27.264) (26.8191, 27.2732) (26.8276, 27.2824) (26.8361, 27.2917) (26.8447, 27.301) (26.8532, 27.3104) (26.8618, 27.3197) (26.8703, 27.3291) (26.8789, 27.3386) (26.8875, 27.3481) (26.8961, 27.3576) (26.9047, 27.3671) (26.9133, 27.3767) (26.9219, 27.3863) (26.9305, 27.396) (26.9392, 27.4057) (26.9478, 27.4154) (26.9565, 27.4252) (26.9651, 27.435) (26.9738, 27.4448) (26.9825, 27.4547) (26.9912, 27.4646) (26.9999, 27.4745) (27.0086, 27.4845) (27.0173, 27.4945) (27.026, 27.5045) (27.0347, 27.5146) (27.0435, 27.5247) (27.0522, 27.5349) (27.061, 27.545) (27.0697, 27.5553) (27.0767, 27.5635) (27.082, 27.5696) (27.0855, 27.5737) (27.0873, 27.5758) knots 0 0 0 0 0 0 0.00416667 0.00833333 0.0125 0.01666667 0.02083333 0.025 0.02916667 0.03333333 0.0375 0.04166667 0.04583333 0.05 0.05416667 0.05833333 0.0625 0.06666667 0.07083333 0.075 0.07916667 0.08333333 0.0875 0.09166667 0.09583333 0.1 0.10416667 0.10833333 0.1125 0.11666667 0.12083333 0.125 0.12916667 0.13333333 0.1375 0.14166667 0.14583333 0.15 0.15416667 0.15833333 0.1625 0.16666667 0.17083333 0.175 0.17916667 0.18333333 0.1875 0.19166667 0.19583333 0.2 0.20416667 0.20833333 0.2125 0.21666667 0.22083333 0.225 0.22916667 0.23333333 0.2375 0.24166667 0.24583333 0.25 0.25416667 0.25833333 0.2625 0.26666667 0.27083333 0.275 0.27916667 0.28333333 0.2875 0.29166667 0.29583333 0.3 0.30416667 0.30833333 0.3125 0.31666667 0.32083333 0.325 0.32916667 0.33333333 0.3375 0.34166667 0.34583333 0.35 0.35416667 0.35833333 0.3625 0.36666667 0.37083333 0.375 0.37916667 0.38333333 0.3875 0.39166667 0.39583333 0.4 0.40416667 0.40833333 0.4125 0.41666667 0.42083333 0.425 0.42916667 0.43333333 0.4375 0.44166667 0.44583333 0.45 0.45416667 0.45833333 0.4625 0.46666667 0.47083333 0.475 0.47916667 0.48333333 0.4875 0.49166667 0.49583333 0.5 0.50416667 0.50833333 0.5125 0.51666667 0.52083333 0.525 0.52916667 0.53333333 0.5375 0.54166667 0.54583333 0.55 0.55416667 0.55833333 0.5625 0.56666667 0.57083333 0.575 0.57916667 0.58333333 0.5875 0.59166667 0.59583333 0.6 0.60416667 0.60833333 0.6125 0.61666667 0.62083333 0.625 0.62916667 0.63333333 0.6375 0.64166667 0.64583333 0.65 0.65416667 0.65833333 0.6625 0.66666667 0.67083333 0.675 0.67916667 0.68333333 0.6875 0.69166667 0.69583333 0.7 0.70416667 0.70833333 0.7125 0.71666667 0.72083333 0.725 0.72916667 0.73333333 0.7375 0.74166667 0.74583333 0.75 0.75416667 0.75833333 0.7625 0.76666667 0.77083333 0.775 0.77916667 0.78333333 0.7875 0.79166667 0.79583333 0.8 0.80416667 0.80833333 0.8125 0.81666667 0.82083333 0.825 0.82916667 0.83333333 0.8375 0.84166667 0.84583333 0.85 0.85416667 0.85833333 0.8625 0.86666667 0.87083333 0.875 0.87916667 0.88333333 0.8875 0.89166667 0.89583333 0.9 0.90416667 0.90833333 0.9125 0.91666667 0.92083333 0.925 0.92916667 0.93333333 0.9375 0.94166667 0.94583333 0.95 0.95416667 0.95833333 0.9625 0.96666667 0.97083333 0.975 0.97916667 0.98333333 0.9875 0.99166667 0.99583333 1 1 1 1 1 1
  line L219 (-10.9662, -14.3955) -> (-10.9659, -14.3948)
  line L220 (20.9569, -7.6094) -> (20.9575, -7.61)
  spline S99 degree 5 poles (26.8955, 23.4662) (26.8956, 23.4662) (26.8958, 23.4663) (26.8961, 23.4664) (26.8966, 23.4666) (26.8973, 23.4669) (26.8981, 23.4672) (26.899, 23.4676) (26.9, 23.4681) (26.9011, 23.4685) (26.9023, 23.4691) (26.9036, 23.4696) (26.905, 23.4702) (26.9065, 23.4709) (26.908, 23.4716) (26.9097, 23.4724) (26.9115, 23.4731) (26.9134, 23.474) (26.9153, 23.4749) (26.9173, 23.4758) (26.9195, 23.4768) (26.9217, 23.4778) (26.924, 23.4788) (26.9263, 23.4799) (26.9288, 23.4811) (26.9313, 23.4823) (26.9339, 23.4835) (26.9366, 23.4848) (26.9394, 23.4861) (26.9423, 23.4875) (26.9452, 23.4889) (26.9482, 23.4903) (26.9513, 23.4918) (26.9544, 23.4934) (26.9577, 23.4949) (26.961, 23.4966) (26.9643, 23.4982) (26.9678, 23.4999) (26.9713, 23.5017) (26.9748, 23.5035) (26.9785, 23.5053) (26.9822, 23.5072) (26.986, 23.5091) (26.9898, 23.5111) (26.9937, 23.5131) (26.9977, 23.5151) (27.0017, 23.5172) (27.0058, 23.5193) (27.01, 23.5215) (27.0142, 23.5237) (27.0185, 23.5259) (27.0228, 23.5282) (27.0272, 23.5306) (27.0317, 23.5329) (27.0362, 23.5353) (27.0408, 23.5378) (27.0454, 23.5403) (27.0501, 23.5428) (27.0549, 23.5454) (27.0597, 23.548) (27.0645, 23.5507) (27.0694, 23.5534) (27.0744, 23.5561) (27.0794, 23.5589) (27.0845, 23.5617) (27.0896, 23.5646) (27.0948, 23.5675) (27.1, 23.5704) (27.1053, 23.5734) (27.1106, 23.5764) (27.116, 23.5795) (27.1214, 23.5826) (27.1269, 23.5857) (27.1324, 23.5889) (27.138, 23.5921) (27.1436, 23.5954) (27.1493, 23.5987) (27.155, 23.602) (27.1608, 23.6054) (27.1666, 23.6088) (27.1725, 23.6123) (27.1784, 23.6158) (27.1843, 23.6193) (27.1903, 23.6229) (27.1963, 23.6265) (27.2024, 23.6301) (27.2085, 23.6338) (27.2147, 23.6376) (27.2209, 23.6413) (27.2271, 23.6451) (27.2334, 23.649) (27.2397, 23.6529) (27.2461, 23.6568) (27.2525, 23.6608) (27.259, 23.6648) (27.2654, 23.6688) (27.272, 23.6729) (27.2785, 23.677) (27.2851, 23.6812) (27.2918, 23.6854) (27.2985, 23.6896) (27.3052, 23.6939) (27.3119, 23.6982) (27.3187, 23.7025) (27.3256, 23.7069) (27.3324, 23.7113) (27.3393, 23.7158) (27.3463, 23.7203) (27.3533, 23.7248) (27.3603, 23.7294) (27.3673, 23.734) (27.3744, 23.7387) (27.3815, 23.7434) (27.3887, 23.7481) (27.3958, 23.7529) (27.4031, 23.7577) (27.4103, 23.7625) (27.4176, 23.7674) (27.4249, 23.7723) (27.4323, 23.7773) (27.4396, 23.7823) (27.447, 23.7873) (27.4545, 23.7924) (27.462, 23.7975) (27.4695, 23.8026) (27.477, 23.8078) (27.4846, 23.813) (27.4922, 23.8183) (27.4998, 23.8235) (27.5074, 23.8289) (27.5151, 23.8342) (27.5228, 23.8396) (27.5306, 23.8451) (27.5384, 23.8506) (27.5462, 23.8561) (27.554, 23.8616) (27.5618, 23.8672) (27.5697, 23.8728) (27.5776, 23.8785) (27.5856, 23.8842) (27.5936, 23.8899) (27.6015, 23.8957) (27.6096, 23.9015) (27.6176, 23.9074) (27.6257, 23.9132) (27.6338, 23.9192) (27.6419, 23.9251) (27.6501, 23.9311) (27.6582, 23.9371) (27.6665, 23.9432) (27.6747, 23.9493) (27.6829, 23.9554) (27.6912, 23.9616) (27.6995, 23.9678) (27.7078, 23.9741) (27.7162, 23.9803) (27.7246, 23.9867) (27.733, 23.993) (27.7414, 23.9994) (27.7498, 24.0058) (27.7583, 24.0123) (27.7668, 24.0188) (27.7753, 24.0253) (27.7838, 24.0319) (27.7924, 24.0385) (27.801, 24.0452) (27.8096, 24.0518) (27.8182, 24.0585) (27.8268, 24.0653) (27.8355, 24.0721) (27.8442, 24.0789) (27.8529, 24.0858) (27.8616, 24.0927) (27.8704, 24.0996) (27.8791, 24.1065) (27.8879, 24.1135) (27.8967, 24.1206) (27.9055, 24.1276) (27.9144, 24.1348) (27.9233, 24.1419) (27.9322, 24.1491) (27.9411, 24.1563) (27.95, 24.1635) (27.9589, 24.1708) (27.9679, 24.1781) (27.9769, 24.1855) (27.9859, 24.1929) (27.9949, 24.2003) (28.0039, 24.2078) (28.013, 24.2153) (28.0221, 24.2228) (28.0312, 24.2303) (28.0403, 24.2379) (28.0494, 24.2456) (28.0585, 24.2532) (28.0677, 24.2609) (28.0769, 24.2687) (28.0861, 24.2765) (28.0953, 24.2843) (28.1045, 24.2921) (28.1137, 24.3) (28.123, 24.3079) (28.1323, 24.3158) (28.1416, 24.3238) (28.1509, 24.3318) (28.1602, 24.3399) (28.1695, 24.348) (28.1789, 24.3561) (28.1882, 24.3643) (28.1976, 24.3724) (28.207, 24.3807) (28.2164, 24.3889) (28.2259, 24.3972) (28.2353, 24.4055) (28.2447, 24.4139) (28.2542, 24.4223) (28.2637, 24.4307) (28.2732, 24.4392) (28.2827, 24.4477) (28.2922, 24.4562) (28.3018, 24.4648) (28.3113, 24.4734) (28.3209, 24.482) (28.3305, 24.4907) (28.34, 24.4994) (28.3496, 24.5081) (28.3593, 24.5169) (28.3689, 24.5257) (28.3785, 24.5345) (28.3882, 24.5434) (28.3978, 24.5523) (28.4075, 24.5613) (28.4172, 24.5702) (28.4269, 24.5792) (28.4366, 24.5883) (28.4464, 24.5973) (28.4561, 24.6065) (28.4658, 24.6156) (28.4756, 24.6248) (28.4854, 24.634) (28.4951, 24.6432) (28.503, 24.6506) (28.5089, 24.6562) (28.5128, 24.66) (28.5147, 24.6618) knots 0 0 0 0 0 0 0.00416667 0.00833333 0.0125 0.01666667 0.02083333 0.025 0.02916667 0.03333333 0.0375 0.04166667 0.04583333 0.05 0.05416667 0.05833333 0.0625 0.06666667 0.07083333 0.075 0.07916667 0.08333333 0.0875 0.09166667 0.09583333 0.1 0.10416667 0.10833333 0.1125 0.11666667 0.12083333 0.125 0.12916667 0.13333333 0.1375 0.14166667 0.14583333 0.15 0.15416667 0.15833333 0.1625 0.16666667 0.17083333 0.175 0.17916667 0.18333333 0.1875 0.19166667 0.19583333 0.2 0.20416667 0.20833333 0.2125 0.21666667 0.22083333 0.225 0.22916667 0.23333333 0.2375 0.24166667 0.24583333 0.25 0.25416667 0.25833333 0.2625 0.26666667 0.27083333 0.275 0.27916667 0.28333333 0.2875 0.29166667 0.29583333 0.3 0.30416667 0.30833333 0.3125 0.31666667 0.32083333 0.325 0.32916667 0.33333333 0.3375 0.34166667 0.34583333 0.35 0.35416667 0.35833333 0.3625 0.36666667 0.37083333 0.375 0.37916667 0.38333333 0.3875 0.39166667 0.39583333 0.4 0.40416667 0.40833333 0.4125 0.41666667 0.42083333 0.425 0.42916667 0.43333333 0.4375 0.44166667 0.44583333 0.45 0.45416667 0.45833333 0.4625 0.46666667 0.47083333 0.475 0.47916667 0.48333333 0.4875 0.49166667 0.49583333 0.5 0.50416667 0.50833333 0.5125 0.51666667 0.52083333 0.525 0.52916667 0.53333333 0.5375 0.54166667 0.54583333 0.55 0.55416667 0.55833333 0.5625 0.56666667 0.57083333 0.575 0.57916667 0.58333333 0.5875 0.59166667 0.59583333 0.6 0.60416667 0.60833333 0.6125 0.61666667 0.62083333 0.625 0.62916667 0.63333333 0.6375 0.64166667 0.64583333 0.65 0.65416667 0.65833333 0.6625 0.66666667 0.67083333 0.675 0.67916667 0.68333333 0.6875 0.69166667 0.69583333 0.7 0.70416667 0.70833333 0.7125 0.71666667 0.72083333 0.725 0.72916667 0.73333333 0.7375 0.74166667 0.74583333 0.75 0.75416667 0.75833333 0.7625 0.76666667 0.77083333 0.775 0.77916667 0.78333333 0.7875 0.79166667 0.79583333 0.8 0.80416667 0.80833333 0.8125 0.81666667 0.82083333 0.825 0.82916667 0.83333333 0.8375 0.84166667 0.84583333 0.85 0.85416667 0.85833333 0.8625 0.86666667 0.87083333 0.875 0.87916667 0.88333333 0.8875 0.89166667 0.89583333 0.9 0.90416667 0.90833333 0.9125 0.91666667 0.92083333 0.925 0.92916667 0.93333333 0.9375 0.94166667 0.94583333 0.95 0.95416667 0.95833333 0.9625 0.96666667 0.97083333 0.975 0.97916667 0.98333333 0.9875 0.99166667 0.99583333 1 1 1 1 1 1
  line L221 (-22.7115, 30.1281) -> (-22.9441, 30.3086)
  line L222 (18.5501, -9.4649) -> (18.7401, -9.6898)
  line L223 (18.7401, -9.6898) -> (18.7406, -9.6904)
  line L224 (20.11, -8.4575) -> (20.1094, -8.4569)
  line L225 (20.7445, -7.4055) -> (20.9569, -7.6094)
  line L226 (-12.5209, -13.3803) -> (-12.6491, -13.6453)
  line L227 (-10.9659, -14.3948) -> (-10.8547, -14.1221)
  spline S100 degree 5 poles (26.5997, 28.4204) (26.597, 28.4199) (26.5917, 28.4189) (26.5837, 28.4174) (26.5731, 28.4154) (26.5599, 28.413) (26.5467, 28.4105) (26.5335, 28.408) (26.5204, 28.4055) (26.5073, 28.4029) (26.4943, 28.4004) (26.4812, 28.3979) (26.4682, 28.3953) (26.4553, 28.3927) (26.4424, 28.3902) (26.4295, 28.3876) (26.4166, 28.385) (26.4038, 28.3824) (26.391, 28.3798) (26.3783, 28.3771) (26.3656, 28.3745) (26.3529, 28.3719) (26.3403, 28.3692) (26.3276, 28.3666) (26.3151, 28.3639) (26.3025, 28.3612) (26.29, 28.3585) (26.2776, 28.3558) (26.2651, 28.3531) (26.2528, 28.3504) (26.2404, 28.3477) (26.2281, 28.3449) (26.2158, 28.3422) (26.2035, 28.3394) (26.1913, 28.3367) (26.1792, 28.3339) (26.167, 28.3311) (26.1549, 28.3283) (26.1428, 28.3255) (26.1308, 28.3227) (26.1188, 28.3199) (26.1069, 28.3171) (26.095, 28.3143) (26.0831, 28.3115) (26.0712, 28.3086) (26.0594, 28.3058) (26.0477, 28.3029) (26.0359, 28.3001) (26.0242, 28.2972) (26.0126, 28.2943) (26.001, 28.2914) (25.9894, 28.2886) (25.9778, 28.2857) (25.9663, 28.2828) (25.9549, 28.2798) (25.9435, 28.2769) (25.9321, 28.274) (25.9207, 28.2711) (25.9094, 28.2682) (25.8982, 28.2652) (25.8869, 28.2623) (25.8757, 28.2593) (25.8646, 28.2564) (25.8535, 28.2534) (25.8424, 28.2504) (25.8314, 28.2475) (25.8204, 28.2445) (25.8094, 28.2415) (25.7985, 28.2385) (25.7877, 28.2355) (25.7768, 28.2325) (25.766, 28.2295) (25.7553, 28.2265) (25.7446, 28.2235) (25.7339, 28.2205) (25.7233, 28.2175) (25.7127, 28.2145) (25.7022, 28.2114) (25.6917, 28.2084) (25.6812, 28.2054) (25.6708, 28.2023) (25.6604, 28.1993) (25.6501, 28.1963) (25.6398, 28.1932) (25.6296, 28.1902) (25.6194, 28.1871) (25.6092, 28.1841) (25.5991, 28.181) (25.589, 28.1779) (25.579, 28.1749) (25.569, 28.1718) (25.559, 28.1688) (25.5491, 28.1657) (25.5393, 28.1626) (25.5294, 28.1596) (25.5197, 28.1565) (25.5099, 28.1534) (25.5003, 28.1503) (25.4906, 28.1473) (25.481, 28.1442) (25.4715, 28.1411) (25.462, 28.138) (25.4525, 28.135) (25.4431, 28.1319) (25.4337, 28.1288) (25.4244, 28.1257) (25.4151, 28.1227) (25.4059, 28.1196) (25.3967, 28.1165) (25.3876, 28.1134) (25.3785, 28.1104) (25.3694, 28.1073) (25.3604, 28.1042) (25.3515, 28.1012) (25.3426, 28.0981) (25.3337, 28.095) (25.3249, 28.092) (25.3161, 28.0889) (25.3074, 28.0859) (25.2988, 28.0828) (25.2901, 28.0798) (25.2816, 28.0767) (25.2731, 28.0737) (25.2646, 28.0706) (25.2562, 28.0676) (25.2478, 28.0645) (25.2394, 28.0615) (25.2312, 28.0585) (25.2229, 28.0555) (25.2148, 28.0524) (25.2066, 28.0494) (25.1986, 28.0464) (25.1905, 28.0434) (25.1826, 28.0404) (25.1746, 28.0374) (25.1668, 28.0344) (25.1589, 28.0315) (25.1512, 28.0285) (25.1434, 28.0255) (25.1358, 28.0226) (25.1282, 28.0196) (25.1206, 28.0166) (25.1131, 28.0137) (25.1056, 28.0108) (25.0982, 28.0078) (25.0909, 28.0049) (25.0836, 28.002) (25.0763, 27.9991) (25.0691, 27.9962) (25.062, 27.9933) (25.0549, 27.9905) (25.0479, 27.9876) (25.0409, 27.9848) (25.034, 27.9819) (25.0271, 27.9791) (25.0203, 27.9762) (25.0136, 27.9734) (25.0069, 27.9706) (25.0002, 27.9678) (24.9936, 27.9651) (24.9871, 27.9623) (24.9806, 27.9595) (24.9742, 27.9568) (24.9679, 27.9541) (24.9616, 27.9514) (24.9553, 27.9486) (24.9492, 27.946) (24.943, 27.9433) (24.937, 27.9406) (24.931, 27.938) (24.925, 27.9353) (24.9192, 27.9327) (24.9133, 27.9301) (24.9076, 27.9275) (24.9019, 27.925) (24.8962, 27.9224) (24.8907, 27.9199) (24.8852, 27.9174) (24.8797, 27.9149) (24.8743, 27.9124) (24.869, 27.9099) (24.8637, 27.9075) (24.8585, 27.905) (24.8534, 27.9026) (24.8483, 27.9002) (24.8433, 27.8979) (24.8384, 27.8955) (24.8335, 27.8932) (24.8287, 27.8909) (24.8239, 27.8886) (24.8193, 27.8863) (24.8147, 27.8841) (24.8101, 27.8819) (24.8056, 27.8797) (24.8012, 27.8775) (24.7969, 27.8754) (24.7926, 27.8733) (24.7884, 27.8712) (24.7843, 27.8691) (24.7802, 27.8671) (24.7763, 27.8651) (24.7723, 27.8631) (24.7685, 27.8611) (24.7647, 27.8592) (24.761, 27.8573) (24.7574, 27.8554) (24.7539, 27.8536) (24.7504, 27.8518) (24.747, 27.85) (24.7437, 27.8482) (24.7404, 27.8465) (24.7372, 27.8449) (24.7341, 27.8432) (24.7311, 27.8416) (24.7282, 27.84) (24.7253, 27.8385) (24.7225, 27.837) (24.7198, 27.8355) (24.7172, 27.8341) (24.7147, 27.8327) (24.7122, 27.8313) (24.7099, 27.83) (24.7076, 27.8287) (24.7054, 27.8275) (24.7033, 27.8263) (24.7012, 27.8252) (24.6993, 27.8241) (24.6974, 27.823) (24.6956, 27.822) (24.694, 27.821) (24.6924, 27.8201) (24.6909, 27.8193) (24.6895, 27.8184) (24.6881, 27.8177) (24.6869, 27.8169) (24.6858, 27.8163) (24.6848, 27.8157) (24.6838, 27.8151) (24.683, 27.8146) (24.6822, 27.8142) (24.6816, 27.8138) (24.6812, 27.8135) (24.6809, 27.8133) (24.6807, 27.8132) (24.6806, 27.8132) knots -1 -1 -1 -1 -1 -1 -0.99583333 -0.99166667 -0.9875 -0.98333333 -0.97916667 -0.975 -0.97083333 -0.96666667 -0.9625 -0.95833333 -0.95416667 -0.95 -0.94583333 -0.94166667 -0.9375 -0.93333333 -0.92916667 -0.925 -0.92083333 -0.91666667 -0.9125 -0.90833333 -0.90416667 -0.9 -0.89583333 -0.89166667 -0.8875 -0.88333333 -0.87916667 -0.875 -0.87083333 -0.86666667 -0.8625 -0.85833333 -0.85416667 -0.85 -0.84583333 -0.84166667 -0.8375 -0.83333333 -0.82916667 -0.825 -0.82083333 -0.81666667 -0.8125 -0.80833333 -0.80416667 -0.8 -0.79583333 -0.79166667 -0.7875 -0.78333333 -0.77916667 -0.775 -0.77083333 -0.76666667 -0.7625 -0.75833333 -0.75416667 -0.75 -0.74583333 -0.74166667 -0.7375 -0.73333333 -0.72916667 -0.725 -0.72083333 -0.71666667 -0.7125 -0.70833333 -0.70416667 -0.7 -0.69583333 -0.69166667 -0.6875 -0.68333333 -0.67916667 -0.675 -0.67083333 -0.66666667 -0.6625 -0.65833333 -0.65416667 -0.65 -0.64583333 -0.64166667 -0.6375 -0.63333333 -0.62916667 -0.625 -0.62083333 -0.61666667 -0.6125 -0.60833333 -0.60416667 -0.6 -0.59583333 -0.59166667 -0.5875 -0.58333333 -0.57916667 -0.575 -0.57083333 -0.56666667 -0.5625 -0.55833333 -0.55416667 -0.55 -0.54583333 -0.54166667 -0.5375 -0.53333333 -0.52916667 -0.525 -0.52083333 -0.51666667 -0.5125 -0.50833333 -0.50416667 -0.5 -0.49583333 -0.49166667 -0.4875 -0.48333333 -0.47916667 -0.475 -0.47083333 -0.46666667 -0.4625 -0.45833333 -0.45416667 -0.45 -0.44583333 -0.44166667 -0.4375 -0.43333333 -0.42916667 -0.425 -0.42083333 -0.41666667 -0.4125 -0.40833333 -0.40416667 -0.4 -0.39583333 -0.39166667 -0.3875 -0.38333333 -0.37916667 -0.375 -0.37083333 -0.36666667 -0.3625 -0.35833333 -0.35416667 -0.35 -0.34583333 -0.34166667 -0.3375 -0.33333333 -0.32916667 -0.325 -0.32083333 -0.31666667 -0.3125 -0.30833333 -0.30416667 -0.3 -0.29583333 -0.29166667 -0.2875 -0.28333333 -0.27916667 -0.275 -0.27083333 -0.26666667 -0.2625 -0.25833333 -0.25416667 -0.25 -0.24583333 -0.24166667 -0.2375 -0.23333333 -0.22916667 -0.225 -0.22083333 -0.21666667 -0.2125 -0.20833333 -0.20416667 -0.2 -0.19583333 -0.19166667 -0.1875 -0.18333333 -0.17916667 -0.175 -0.17083333 -0.16666667 -0.1625 -0.15833333 -0.15416667 -0.15 -0.14583333 -0.14166667 -0.1375 -0.13333333 -0.12916667 -0.125 -0.12083333 -0.11666667 -0.1125 -0.10833333 -0.10416667 -0.1 -0.09583333 -0.09166667 -0.0875 -0.08333333 -0.07916667 -0.075 -0.07083333 -0.06666667 -0.0625 -0.05833333 -0.05416667 -0.05 -0.04583333 -0.04166667 -0.0375 -0.03333333 -0.02916667 -0.025 -0.02083333 -0.01666667 -0.0125 -0.00833333 -0.00416667 0 0 0 0 0 0